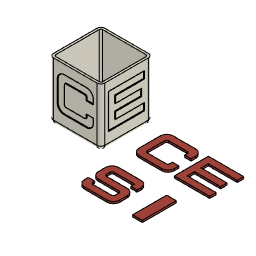
Ceis_porta_penne (Autodesk Fusion 360 design; units mm, degrees)
Autodesk Fusion 360 part; units mm, degrees
sketch "Schizzo1" plane through (0, 0, 0) normal (0, 0, 1) x (1, 0, 0)
  line L0 (0, 0) -> (80, 0)
  line L1 (80, 0) -> (80, 80)
  line L2 (80, 80) -> (0, 80)
  line L3 (0, 80) -> (0, 0)
  dimension "d1" = 80
  dimension "d2" = 80
  constraint horizontal L0
  constraint vertical L1
  constraint horizontal L2
  constraint vertical L3
  constraint coincident L0.start L3.end
  measures "d1" distance of L1.end L2.end
  measures "d2" distance of L0.start L2.end
extrude "Estrusione1" add sketch "Schizzo1" along normal blind 90 makes body 1
fillet "Raccordo1" radius 6 8 edges at (0, 0, 45) (80, 0, 45) (80, 80, 45) (80, 40, 0) (40, 0, 0) (0, 80, 45) (40, 80, 0) (0, 40, 0) on bodies 1
sketch "Schizzo2" plane through (0, 0, 0) normal (0, -1, 0) x (1, 0, 0)
  line L0 (74, 90) -> (6, 90)
  line L1 (6, 6) -> (74, 6)
  line L2 (74, 90) -> (74, 6)
  line L3 (25.5, 32.5) -> (54.5, 32.5)
  arc A0 (54.5, 32.5) -> (57, 35) centre (54.5, 35) ccw
  line L4 (57, 39.5) -> (57, 35)
  line L5 (57, 39.5) -> (68, 39.5)
  line L6 (68, 32) -> (68, 39.5)
  arc A1 (57.5, 21.5) -> (68, 32) centre (57.5, 32) ccw
  line L7 (22.5, 21.5) -> (57.5, 21.5)
  arc A2 (12, 32) -> (22.5, 21.5) centre (22.5, 32) ccw
  line L8 (12, 65) -> (12, 32)
  arc A3 (22.5, 75.5) -> (12, 65) centre (22.5, 65) ccw
  line L9 (57.5, 75.5) -> (22.5, 75.5)
  arc A4 (68, 65) -> (57.5, 75.5) centre (57.5, 65) ccw
  line L10 (68, 57.5) -> (68, 65)
  line L11 (57, 57.5) -> (68, 57.5)
  line L12 (57, 62) -> (57, 57.5)
  arc A5 (57, 62) -> (54.5, 64.5) centre (54.5, 62) ccw
  line L13 (25.5, 64.5) -> (54.5, 64.5)
  arc A6 (25.5, 64.5) -> (23, 62) centre (25.5, 62) ccw
  line L14 (23, 62) -> (23, 35)
  arc A7 (23, 35) -> (25.5, 32.5) centre (25.5, 35) ccw
  constraint tangent L3 A7
  constraint tangent A6 L14
  constraint tangent L3 A0
  constraint tangent L9 A4
  constraint tangent A0 L4
  constraint tangent L6 A1
  constraint tangent A2 L8
  constraint tangent L8 A3
  constraint tangent A3 L9
  constraint tangent A4 L10
  constraint tangent L12 A5
  constraint tangent A5 L13
  constraint tangent L13 A6
  constraint tangent L14 A7
sketch "Schizzo4" plane through (80, 0, 0) normal (1, 0, 0) x (0, 1, 0)
  line L0 (6, 90) -> (6, 6)
  line L1 (6, 6) -> (74, 6)
  line L2 (74, 6) -> (74, 90)
  line L3 (74, 90) -> (6, 90)
  line L4 (23, 64.5) -> (68, 64.5)
  line L5 (23, 54) -> (23, 64.5)
  line L6 (23, 54) -> (63.5383, 54)
  line L7 (63.5383, 43) -> (63.5383, 54)
  line L8 (23, 43) -> (63.5383, 43)
  line L9 (23, 32.5) -> (23, 43)
  line L10 (23, 32.5) -> (68, 32.5)
  line L11 (12, 21.5) -> (68, 21.5)
  line L12 (12, 21.5) -> (12, 48.5)
  line L13 (12, 75.5) -> (12, 48.5)
  line L14 (68, 75.5) -> (68, 64.5)
  line L15 (12, 75.5) -> (68, 75.5)
  line L16 (68, 21.5) -> (68, 32.5)
sketch "Schizzo5" plane through (0, 80, 0) normal (0, 1, 0) x (-1, 0, 0)
  line L0 (-74, 90) -> (-74, 6)
  line L1 (-74, 6) -> (-6, 6)
  line L2 (-6, 6) -> (-6, 90)
  line L3 (-6, 90) -> (-74, 90)
  line L4 (0, 6) -> (0, 90)
  line L5 (-48, 46.9583) -> (-48, 75.4715)
  line L6 (-48, 75.4715) -> (-32, 75.4715)
  line L7 (-32, 75.4715) -> (-32, 48.4858)
  line L8 (-48, 50.0133) -> (-48, 21.5)
  line L9 (-48, 21.5) -> (-32, 21.5)
  line L10 (-32, 21.5) -> (-32, 48.4858)
sketch "Schizzo6" plane through (0, 0, 0) normal (-1, 0, 0) x (0, -1, 0)
  line L0 (-6, 6) -> (-6, 90)
  line L1 (-6, 90) -> (-74, 90)
  line L2 (-74, 90) -> (-74, 6)
  line L3 (-74, 6) -> (-6, 6)
  line L4 (-67.5, 75) -> (-67.2838, 75)
  line L5 (-57.5, 75) -> (-57.5, 74.8995)
  line L6 (-67.5, 65) -> (-67.3995, 65)
  arc A0 (-12, 64.9982) -> (-22.5, 75.5) centre (-22.5, 65) ccw
  line L7 (-22.5, 75.5) -> (-58, 75.5)
  line L8 (-58, 75.5) -> (-58, 75.3875)
  line L9 (-68, 65.5) -> (-67.8875, 65.5)
  line L10 (-68, 65.5) -> (-68, 53.4975)
  arc A1 (-12, 43.4968) -> (-22.5, 54) centre (-22.5, 43.5) ccw
  line L11 (-22.5, 54) -> (-54.5, 54)
  arc A2 (-57, 56.5) -> (-54.5, 54) centre (-54.5, 56.5) ccw
  line L12 (-57, 62) -> (-57, 56.5)
  arc A3 (-54.5, 64.5) -> (-57, 62) centre (-54.5, 62) ccw
  line L13 (-54.5, 64.5) -> (-25.5, 64.5)
  arc A4 (-23, 62) -> (-25.5, 64.5) centre (-25.5, 62) ccw
  line L14 (-23, 58.5) -> (-23, 62)
  line L15 (-23, 58.5) -> (-12, 58.5)
  line L16 (-12, 58.5) -> (-12, 65.0017)
  arc A5 (-68, 53.5026) -> (-57.5, 43) centre (-57.5, 53.5) ccw
  line L17 (-57.5, 43) -> (-25.5, 43)
  arc A6 (-23, 40.5) -> (-25.5, 43) centre (-25.5, 40.5) ccw
  line L18 (-23, 35) -> (-23, 40.5)
  arc A7 (-25.5, 32.5) -> (-23, 35) centre (-25.5, 35) ccw
  line L19 (-54.5, 32.5) -> (-25.5, 32.5)
  arc A8 (-57, 35) -> (-54.5, 32.5) centre (-54.5, 35) ccw
  line L20 (-57, 38.5) -> (-57, 35)
  line L21 (-68, 38.5) -> (-57, 38.5)
  line L22 (-68, 38.5) -> (-68, 32)
  arc A9 (-68, 32) -> (-57.5, 21.5) centre (-57.5, 32) ccw
  line L23 (-57.5, 21.5) -> (-22.5, 21.5)
  arc A10 (-22.5, 21.5) -> (-12, 32.0018) centre (-22.5, 32) ccw
  line L24 (-12, 31.9983) -> (-12, 43.503)
  arc A11 (-58, 75.5) -> (-68, 65.5) centre (-58, 65.5) ccw
  constraint tangent L17 A6
  constraint tangent L22 A9
  constraint tangent L19 A8
  constraint tangent A5 L17
  constraint tangent A8 L20
  constraint tangent A7 L19
  constraint tangent A9 L23
  constraint tangent L23 A10
  constraint tangent A1 L11
  constraint tangent A3 L13
  constraint tangent L11 A2
  constraint tangent L13 A4
  constraint parallel L5 L8
  constraint parallel L6 L9
  constraint tangent A0 L7
  constraint tangent L10 A11
sketch "Schizzo8" plane through (0, 0, 90) normal (0, 0, 1) x (-1, 0, 0)
  arc A0 (-74, 0) -> (-80, -6) centre (-74, -6) ccw
  line L0 (-80, -6) -> (-80, -74)
  arc A1 (-80, -74) -> (-74, -80) centre (-74, -74) ccw
  line L1 (-74, -80) -> (-6, -80)
  arc A2 (-6, -80) -> (0, -74) centre (-6, -74) ccw
  line L2 (0, -74) -> (0, -6)
  arc A3 (0, -6) -> (-6, 0) centre (-6, -6) ccw
  line L3 (-6, 0) -> (-74, 0)
  line L4 (-3.5, -74) -> (-3.5, -6)
  arc A4 (-3.5, -6) -> (-6, -3.5) centre (-6, -6) ccw
  line L5 (-6, -3.5) -> (-74, -3.5)
  arc A5 (-74, -3.5) -> (-76.5, -6) centre (-74, -6) ccw
  line L6 (-76.5, -6) -> (-76.5, -74)
  arc A6 (-76.5, -74) -> (-74, -76.5) centre (-74, -74) ccw
  line L7 (-74, -76.5) -> (-6, -76.5)
  arc A7 (-6, -76.5) -> (-3.5, -74) centre (-6, -74) ccw
  dimension "d65" = -3.5
extrude "Estrusione2" cut sketch "Schizzo8" against normal blind 86 contours L4 A4 L5 A5 L6 A6 L7 A7 bodies 1
fillet "Raccordo2" radius 6 8 edges at (76.5, 40, 4) (75.7678, 4.2322, 4) (40, 3.5, 4) (4.2322, 4.2322, 4) (3.5, 40, 4) (4.2322, 75.7678, 4) (40, 76.5, 4) (75.7678, 75.7678, 4) on bodies 1
sketch "Schizzo9" plane through (0, 0, 0) normal (0, 0, 1) x (1, 0, 0)
  arc A0 (117.5, 35) -> (120.5, 32) centre (120.5, 35) ccw
  arc A1 (152.5, 22) -> (162.5, 32) centre (152.5, 32) ccw
  arc A2 (152.5, 62) -> (149.5, 65) centre (149.5, 62) ccw
  line L0 (107.5, 75) -> (107.5, 22)
  arc A3 (149.5, 32) -> (152.5, 35) centre (149.5, 35) ccw
  line L1 (162.5, 22) -> (162.5, 75)
  line L2 (152.5, 75) -> (152.5, 22)
  line L3 (107.5, 22) -> (162.5, 22)
  line L4 (107.5, 65) -> (162.5, 65)
  line L5 (152.5, 35) -> (149.5, 35)
  line L6 (117.5, 75) -> (117.5, 22)
  line L7 (162.5, 75) -> (107.5, 75)
  line L8 (107.5, 32) -> (162.5, 32)
  line L9 (117.5, 32) -> (120.5, 32)
  line L10 (152.5, 39) -> (162.5, 39)
  line L11 (152.5, 58) -> (162.5, 58)
  arc A4 (107.5, 32) -> (117.5, 22) centre (117.5, 32) ccw
  arc A5 (120.5, 65) -> (117.5, 62) centre (120.5, 62) ccw
  arc A6 (162.5, 65) -> (152.5, 75) centre (152.5, 65) ccw
  arc A7 (117.5, 75) -> (107.5, 65) centre (117.5, 65) ccw
  dimension "d70" = 17
  constraint horizontal L3
  constraint vertical L1
  constraint horizontal L7
  constraint vertical L0
  constraint coincident L6.start L7
  constraint coincident L6.end L3
  constraint perpendicular L3 L6
  constraint coincident L2.start L7
  constraint perpendicular L2 L7
  constraint coincident L4.start L0
  constraint coincident L4.end L1
  constraint perpendicular L1 L4
  constraint coincident L8.start L0
  constraint coincident A1.end L1
  constraint perpendicular L1 L8
  constraint coincident A7.centre L6
  constraint coincident A7.centre L4
  constraint coincident A6.centre L4
  constraint coincident A6.centre L2
  constraint coincident L9.start L6
  constraint coincident L9.start L8
  constraint coincident A1.centre L8
  constraint coincident A1.centre L2
  constraint coincident L9.start A4.centre
  constraint perpendicular L6 L9
  constraint tangent A0 L6
  constraint coincident A3.end L2
  constraint perpendicular L2 L5
  constraint coincident A3.centre L5.end
  constraint tangent A2 L4
  constraint coincident A5.end L6
  constraint coincident A5.start L4
  constraint coincident A0.start L6
  constraint coincident A3.start L8
  constraint coincident A2.end L4
  constraint coincident A2.start L2
  constraint coincident L11.end L1
  constraint perpendicular L1 L11
  constraint coincident L11.start L2
  constraint coincident L10.start L2
  constraint coincident L10.end L1
  constraint perpendicular L1 L10
  measures "d70" distance of L3 L10
sketch "Schizzo11" plane through (0, 0, 0) normal (0, 0, 1) x (1, 0, 0)
  line L0 (172.5, 48.5) -> (227.5, 48.5)
  line L1 (227.5, 75) -> (227.5, 65)
  line L2 (227.5, 22) -> (172.5, 22)
  line L3 (227.5, 75) -> (227.5, 22)
  line L4 (172.5, 53.5) -> (227.5, 53.5)
  line L5 (172.5, 22) -> (227.5, 22)
  line L6 (172.5, 43.5) -> (227.5, 43.5)
  line L7 (223.0383, 43.5) -> (223.0383, 53.5)
  line L8 (172.5, 65) -> (227.501, 65)
  line L9 (227.5, 22) -> (227.5, 32)
  line L10 (172.5, 75) -> (227.5, 75)
  line L11 (182.5, 22) -> (182.5, 75)
  line L12 (172.5, 22) -> (172.5, 48.5)
  line L13 (172.5, 75) -> (172.5, 48.5)
  line L14 (172.5, 22) -> (172.5, 75)
  line L15 (172.5, 32) -> (227.5, 32)
  line L16 (172.5, 75) -> (227.5, 75)
  dimension "d71" = -5
  dimension "d72" = 10
  dimension "d73" = 10
  dimension "d74" = 26.5
  dimension "d75" = 5
  constraint perpendicular L5 L9
  constraint perpendicular L5 L12
  constraint horizontal L10
  constraint vertical L3
  constraint horizontal L2
  constraint coincident L11.start L5
  constraint coincident L11.end L10
  constraint perpendicular L10 L11
  constraint horizontal L8
  constraint coincident L8.start L14
  constraint coincident L8.start L13
  constraint coincident L15.start L12
  constraint coincident L15.start L14
  constraint coincident L9.end L3
  constraint perpendicular L3 L15
  constraint coincident L6.start L14
  constraint coincident L6.end L3
  constraint perpendicular L3 L6
  constraint coincident L0.start L14
  constraint coincident L0.end L3
  constraint perpendicular L0 L3
  constraint coincident L7.start L6
  constraint coincident L7.end L4
  constraint perpendicular L4 L7
  measures "d72" distance of L11 L14
  measures "d73" distance of L8 L10
  measures "d74" distance of L0 L10
  measures "d75" distance of L0 L6
sketch "Schizzo14" plane through (0, 0, 0) normal (0, 0, 1) x (1, 0, 0)
  line L0 (152.5, -26) -> (162.5, -26)
  arc A0 (152.5, -63) -> (162.5, -52.9983) centre (152.5, -53) ccw
  arc A1 (149.5, -53) -> (152.5, -50) centre (149.5, -50) ccw
  arc A2 (162.5, -20.0017) -> (152.5, -10) centre (152.5, -20) ccw
  arc A3 (152.5, -23) -> (149.5, -20) centre (149.5, -23) ccw
  line L1 (152.5, -63) -> (152.5, -10)
  line L2 (162.5, -63) -> (162.5, -10)
  arc A4 (162.5, -41.503) -> (152.5, -31.5) centre (152.5, -41.5) ccw
  arc A5 (152.5, -44.5) -> (149.5, -41.5) centre (149.5, -44.5) ccw
  line L3 (107.5, -63) -> (162.5, -63)
  line L4 (117.5, -10) -> (117.5, -63)
  line L5 (107.5, -20) -> (162.5, -20)
  arc A6 (107.5, -53) -> (117.5, -63) centre (117.5, -53) ccw
  line L6 (107.5, -10) -> (107.5, -63)
  line L7 (152.5, -31.5) -> (117.5, -31.5)
  line L8 (107.5, -10) -> (107.7162, -10)
  line L9 (107.5, -47) -> (117.5, -47)
  arc A7 (117.8974, -21.5079) -> (117.5, -21.5) centre (117.5, -31.5) ccw
  arc A8 (107.5, -31.4975) -> (117.5, -41.5) centre (117.5, -31.5) ccw
  arc A9 (117.5, -10.1005) -> (107.6005, -20) centre (117.5, -20) ccw
  arc A10 (152.1026, -51.4921) -> (152.5, -51.5) centre (152.5, -41.5) ccw
  arc A11 (117.5, -28.5) -> (120.5, -31.5) centre (120.5, -28.5) ccw
  line L10 (107.5, -53) -> (162.5, -53)
  arc A12 (117.5, -50) -> (120.5, -53) centre (120.5, -50) ccw
  line L11 (117.5, -41.5) -> (152.5, -41.5)
  arc A13 (120.5, -20) -> (117.5, -23) centre (120.5, -23) ccw
  line L12 (162.5, -10) -> (107.5, -10)
  constraint horizontal L3
  constraint vertical L2
  constraint horizontal L12
  constraint vertical L6
  constraint coincident L5.start L6
  constraint coincident L5.end L2
  constraint perpendicular L2 L5
  constraint coincident A6.start L6
  constraint coincident L10.end L2
  constraint perpendicular L2 L10
  constraint coincident L8.end L12
  constraint coincident L4.start L12
  constraint perpendicular L4 L10
  constraint coincident A0.start L3
  constraint coincident A2.end L12
  constraint perpendicular L1 L12
  constraint coincident A9.centre L4
  constraint coincident A9.centre L5
  constraint coincident A0.centre L1
  constraint coincident A0.centre L10
  constraint coincident A2.centre L1
  constraint coincident A2.centre L5
  constraint coincident L9.start L6
  constraint coincident L9.end L4
  constraint perpendicular L4 L9
  constraint coincident L0.start L1
  constraint coincident L0.end L2
  constraint perpendicular L0 L2
  constraint coincident A9.start L4
  constraint coincident A9.end L5
  constraint coincident A0.end L2
  constraint coincident A2.start L2
  constraint tangent L10 A12
  constraint tangent A3 L5
  constraint tangent L5 A13
  constraint tangent A1 L10
  constraint coincident A13.end L4
  constraint coincident A13.start L5
  constraint coincident A3.end L5
  constraint coincident A3.start L1
  constraint coincident A12.end L10
  constraint coincident A12.start L4
  constraint coincident A1.end L1
  constraint coincident A1.start L10
  constraint coincident A4.end L1
  constraint perpendicular L1 L7
  constraint coincident L7.end L4
  constraint coincident A8.end L4
  constraint coincident A4.centre L1
  constraint perpendicular L1 L11
  constraint tangent L7 A11
  constraint tangent A5 L11
  constraint coincident L7.end A7.centre
  constraint coincident A4.centre A10.centre
  constraint coincident A7.end L4
  constraint coincident A8.start L6
  constraint coincident A7.start A13
  constraint concentric A7 A8
  constraint coincident A10.start A1
  constraint coincident A10.end L1
  constraint coincident A4.start L2
  constraint concentric A4 A10
  constraint coincident A5.end L11
  constraint coincident A5.start L1
  constraint coincident A11.end L7
  constraint coincident A11.start L4
sketch "Schizzo15" plane through (0, 0, 0) normal (0, 0, 1) x (1, 0, 0)
  line L0 (207.5, -10.0285) -> (207.5, -36.5142)
  line L1 (192.5, -10.0285) -> (207.5, -10.0285)
  line L2 (172.5, -63) -> (172.5, -10)
  line L3 (160.0456, -36.5142) -> (222.6571, -36.5142)
  line L4 (192.5, -38.0417) -> (192.5, -10.0285)
  line L5 (172.5, -10) -> (227.5, -10)
  line L6 (227.5, -63) -> (172.5, -63)
  line L7 (166, 5) -> (166, -79)
  line L8 (227.5, -10) -> (227.5, -63)
  line L9 (207.5, -63) -> (207.5, -36.5142)
  line L10 (192.5, -63) -> (207.5, -63)
  line L11 (192.5, -34.9867) -> (192.5, -63)
  dimension "d76" = 15
  constraint parallel L7 L11
  constraint perpendicular L10 L11
  constraint perpendicular L9 L10
  constraint perpendicular L3 L9
  constraint coincident L0.end L3
  constraint symmetric L11.start L4.start L3
  constraint symmetric L10.start L1.start L3
  constraint symmetric L0.start L9.start L3
  constraint symmetric L0.end L9.end L3
  constraint horizontal L5
  constraint vertical L8
  constraint horizontal L6
  constraint vertical L2
  measures "d76" distance of L9.start L10.start
extrude "Estrusione3" cut sketch "Schizzo2" against normal blind 1 bodies 1
extrude "Estrusione4" cut sketch "Schizzo4" against normal blind 1 contours L4 L5 L6 L7 L8 L9 L10 L11 L12 L13 L14 L15 L16 bodies 1
extrude "Estrusione5" cut sketch "Schizzo5" against normal blind 1 contours L5 L6 L7 L8 L9 L10 bodies 1
extrude "Estrusione6" cut sketch "Schizzo6" against normal blind 1 contours A0 L7 L10 A1 L11 A2 L12 A3 L13 A4 L14 L15 L16 A5 L17 A6 L18 A7 L19 A8 L20 L21 L22 A9 L23 A10 L24 A11 bodies 1
extrude "Estrusione7" add sketch "Schizzo9" sketch "Schizzo14" sketch "Schizzo11" sketch "Schizzo15" along normal blind 3 separate body contours L0 L4 L6 L8 | A0 L6 L8 L9 | L2 L3 L6 L8 L9 | L4 L6 A5 | L6 L8 A4 | A3 L2 L8 | L2 L4 L6 L7 | L4 L6 A7 | L1 L2 L8 L10 | A1 L2 L8 | A2 L2 L4 | L2 L4 A6 | L1 L2 L4 L11 of sketch 2 contours L0 L1 L2 L5 | L1 L2 A4 L10 | L1 L4 L7 L11 | A2 L1 L5 | L1 A5 L11 | L4 L7 A11 | L1 L4 L5 L12 | A0 L1 L10 | L4 L5 L6 A8 | L4 L5 A7 A13 | L1 L3 L4 L10 | A1 L1 A10 L10 | A1 L1 A10 | L4 A7 A13 | L4 L5 A9 | L4 A6 L10 | L4 L6 L9 L10 | L4 L10 A12 of sketch 3 contours L0 L4 L11 L13 L14 | L0 L6 L11 L12 L14 | L0 L4 L7 L11 | L0 L6 L7 L11 | L6 L11 L12 L14 L15 | L4 L8 L11 L13 L14 | L2 L5 L11 L12 L14 L15 | L8 L10 L11 L13 L14 L16 | L2 L3 L5 L9 L11 L15 | L1 L3 L8 L10 L11 L16 of sketch 4 contours L0 L1 L3 L4 L11 | L3 L4 L6 L9 L10 L11 makes body 2 at (175.8333, 46.8333, 0) makes body 3 at (139.8333, 71.6667, 0) makes body 4 at (130.1667, -59.6667, 0) makes body 5 at (202.5, -45.3428, 0)
fillet "Raccordo3" radius 0.6 28 edges at (1, 23, 60.25) (1, 23.7322, 63.7678) (1, 40, 64.5) (1, 56.2678, 63.7678) (1, 57, 59.25) (1, 56.2678, 54.7322) (1, 38.5, 54) (1, 15.0765, 50.9257) (1, 12, 37.7507) (1, 15.076, 24.5748) (1, 40, 21.5) (1, 64.9246, 24.5754) (1, 68, 35.25) (1, 62.5, 38.5) (1, 57, 36.75) (1, 56.2678, 33.2322) (1, 40, 32.5) (1, 23.7322, 33.2322) (1, 23, 37.75) (1, 23.7322, 42.2678) (1, 41.5, 43) (1, 64.9256, 46.0763) (1, 68, 59.5013) (1, 65.0711, 72.5711) (1, 40.25, 75.5) (1, 15.076, 72.4252) (1, 12, 61.7509) (1, 17.5, 58.5) on bodies 1
fillet "Raccordo4" radius 0.6 4 edges at (40, 79, 21.5) (48, 79, 48.4858) (40, 79, 75.4715) (32, 79, 48.4858) on bodies 1
fillet "Raccordo5" radius 0.6 12 edges at (79, 23, 37.75) (79, 43.2691, 43) (79, 23, 59.25) (79, 40, 21.5) (79, 68, 27) (79, 63.5383, 48.5) (79, 68, 70) (79, 45.5, 64.5) (79, 12, 48.5) (79, 40, 75.5) (79, 43.2691, 54) (79, 45.5, 32.5) on bodies 1
fillet "Raccordo6" radius 0.6 20 edges at (57, 1, 59.75) (56.2678, 1, 63.7678) (40, 1, 64.5) (23.7322, 1, 63.7678) (23, 1, 48.5) (23.7322, 1, 33.2322) (40, 1, 32.5) (56.2678, 1, 33.2322) (57, 1, 37.25) (62.5, 1, 57.5) (68, 1, 35.75) (64.9246, 1, 24.5754) (40, 1, 21.5) (15.0754, 1, 24.5754) (12, 1, 48.5) (15.0754, 1, 72.4246) (40, 1, 75.5) (64.9246, 1, 72.4246) (68, 1, 61.25) (62.5, 1, 39.5) on bodies 1
named bodies: "portapenne"
